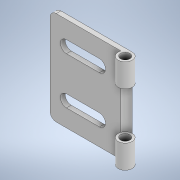
# Autodesk Inventor part: Hinge1
Saved by Autodesk Inventor 2022 (Build 260153000, 153)
## iProperties
Created: 2021-06-15
Part Number: Hinge1
Material: Generic
Document SubType Name: Modeling
Designer: Cornee
Density: 1 g/cm^3
Appearance: Default
Author: Cornee
Autodesk Inventor part; units mm, degrees
ref_plane "YZ Plane" through (0, 0, 0) normal (1, 0, 0) x (0, 1, 0)
ref_plane "XZ Plane" through (0, 0, 0) normal (0, 1, 0) x (-1, 0, 0)
ref_plane "XY Plane" through (0, 0, 0) normal (0, 0, 1) x (1, 0, 0)
sketch "Sketch1" plane through (0, 0, 0) normal (0, 0, 1) x (1, 0, 0)
  line L0 (1.6391, 1.0487) -> (37.6391, 1.0487)
  line L1 (37.6391, 1.0487) -> (37.6391, 41.0487)
  line L2 (37.6391, 41.0487) -> (1.6391, 41.0487)
  line L3 (1.6391, 41.0487) -> (1.6391, 1.0487)
  arc A0 (8.6391, 33.6487) -> (8.6391, 28.4487) centre (8.6391, 31.0487) ccw
  line L4 (8.6391, 31.0487) -> (8.6391, 33.6487) construction
  line L5 (8.6391, 31.0487) -> (11.2391, 31.0487) construction
  line L6 (8.6391, 31.0487) -> (8.6391, 28.4487) construction
  arc A1 (8.6391, 13.6487) -> (8.6391, 8.4487) centre (8.6391, 11.0487) ccw
  line L7 (8.6391, 11.0487) -> (8.6391, 13.6487) construction
  line L8 (8.6391, 11.0487) -> (11.2391, 11.0487) construction
  line L9 (8.6391, 11.0487) -> (8.6391, 8.4487) construction
  arc A2 (22.6391, 28.4487) -> (22.6391, 33.6487) centre (22.6391, 31.0487) ccw
  line L10 (22.6391, 31.0487) -> (22.6391, 33.6487) construction
  line L11 (22.6391, 31.0487) -> (25.2391, 31.0487) construction
  line L12 (22.6391, 31.0487) -> (22.6391, 28.4487) construction
  arc A3 (22.6391, 8.4487) -> (22.6391, 13.6487) centre (22.6391, 11.0487) ccw
  line L13 (22.6391, 11.0487) -> (22.6391, 13.6487) construction
  line L14 (22.6391, 11.0487) -> (25.2391, 11.0487) construction
  line L15 (22.6391, 11.0487) -> (22.6391, 8.4487) construction
  line L16 (8.6391, 33.6487) -> (22.6391, 33.6487)
  line L17 (8.6391, 28.4487) -> (22.6391, 28.4487)
  line L18 (8.6391, 13.6487) -> (22.6391, 13.6487)
  line L19 (8.6391, 8.4487) -> (22.6391, 8.4487)
  point P0 (0, 0)
  point P1 (22.6391, 33.6487)
  dimension "d0" = 36
  dimension "d1" = 40
  dimension "d2" = 2.6
  dimension "d3" = 90
  dimension "d4" = 180
  dimension "d5" = 2.6
  dimension "d6" = 90
  dimension "d7" = 180
  dimension "d8" = 7
  dimension "d9" = 10
  dimension "d10" = 30
  dimension "d11" = 2.6
  dimension "d12" = 90
  dimension "d13" = 180
  dimension "d14" = 2.6
  dimension "d15" = 90
  dimension "d16" = 180
  dimension "d17" = 21
  constraints: 40 end point, 8 point on circle, 6 horizontal, 5 perpendicular, 4 centre point, 2 horizontal alignment, 2 parallel, 2 vertical alignment
  measures "d0" distance of L2.end L1.end
  measures "d1" distance of L1.end L0.end
  measures "d2" radius of A0
  measures "d3" angle of L5 L4
  measures "d4" angle of L4 L6
  measures "d5" radius of A1
  measures "d6" angle of L8 L7
  measures "d7" angle of L7 L9
  measures "d8" distance from line of L3 L7.start
  measures "d9" distance from line of L0 L7.start
  measures "d10" distance from line of L0 L4.start
  measures "d11" radius of A2
  measures "d12" angle of L11 L10
  measures "d13" angle of L10 L12
  measures "d14" radius of A3
  measures "d15" angle of L14 L13
  measures "d16" angle of L13 L15
  measures "d17" distance from line of L3 L10.start
extrude "Extrusion1" add sketch "Sketch1" along normal blind 2
fillet "Fillet1" radius 2.6 1 edges at (1.6391, 41.0487, 1)
fillet "Fillet2" radius 2.6 1 edges at (1.6391, 1.0487, 1)
sketch "Sketch2" plane through (37.6391, 1.0487, 0) normal (0, -1, 0) x (1, 0, 0)
  circle A0 centre (-3, 3) radius 2
  circle A1 centre (-3, 3) radius 3
  line L0 (0, 0) -> (0, 2) projected
  line L1 (-33.4, 0) -> (0, 0) projected
  line L2 (-3, 0) -> (0, 0)
  line L3 (0, 2) -> (-0.1716, 2)
  line L4 (-33.4, 2) -> (0, 2) projected
  line L5 (0, 2) -> (0, 0)
  arc A2 (-3, 0) -> (-0.1716, 2) centre (-3, 3) ccw
  point P0 (-37.6391, 0)
  point P1 (-1.2679, 2)
  point P2 (-4.7321, 2)
  point P3 (-5.8284, 2)
  dimension "d22" = 4
  dimension "d23" = 6
  dimension "d24" = 3
  dimension "d25" = 3
  constraints: 6 end point, 4 point on circle, 3 centre point, 2 coincident, 2 point on line, 1 collinear, 1 perpendicular
  measures "d22" diameter of A0
  measures "d23" diameter of A1
  measures "d24" distance from line of A0.centre L0
  measures "d25" distance from line of A0.centre L1
extrude "Extrusion2" cut sketch "Sketch2" against normal through all contours L3 L0 L1 A1
extrude "Extrusion3" cut sketch "Sketch2" against normal through all contours L4 A0 picked at (-3.228, 1.4585)
extrude "Extrusion4" add sketch "Sketch2" against normal blind 10 contours A0 L4 A1 picked at (-0.3839, 3.4074)
extrude "Extrusion5" add sketch "Sketch2" along normal blind 10 from surface at -40 contours A0 L4 A1 picked at (-0.3839, 3.4074)
extrude "Extrusion6" cut sketch "Sketch2" along normal up to surface (20 mm away) from surface at -30 contours A0 L4 A1 picked at (-5.3533, 1.7803)
body "Solid1"
